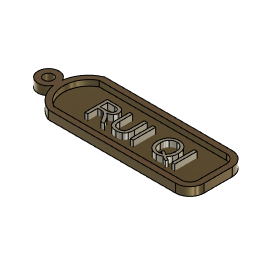
Keychain v1 (Autodesk Fusion 360 design; units mm, degrees)
Autodesk Fusion 360 part; units mm, degrees
sketch "Sketch1" plane through (0, 0, 0) normal (0, 0, 1) x (1, 0, 0) in component "Component"
  line L0 (0, 0) -> (45, 0)
  line L1 (50, 5) -> (50, 15)
  line L2 (45, 20) -> (0, 20)
  arc A0 (50, 15) -> (45, 20) centre (45, 15) ccw
  arc A1 (45, 0) -> (50, 5) centre (45, 5) ccw
  arc A2 (-6.5358, 11.6362) -> (-6.5358, 8.3638) centre (-9.91, 10) ccw
  arc A3 (0, 20) -> (-6.5358, 11.6362) centre (4.1775, 10) ccw
  arc A4 (-6.5358, 8.3638) -> (0, 0) centre (4.1775, 10) ccw
  circle A5 centre (-9.91, 10) radius 1.75
  line L3 (0, 2) -> (45, 2)
  line L4 (48, 5) -> (48, 15)
  line L5 (45, 18) -> (0, 18)
  arc A6 (0, 18) -> (0, 2) centre (4.537, 10) ccw
  arc A7 (45, 2) -> (48, 5) centre (45, 5) ccw
  arc A8 (48, 15) -> (45, 18) centre (45, 15) ccw
  line L6 (7.2298, 5.0727) -> (38.989, 5.0727) construction
  line L7 (38.989, 5.0727) -> (38.989, 16.0727) construction
  line L8 (38.989, 16.0727) -> (7.2298, 16.0727) construction
  line L9 (7.2298, 16.0727) -> (7.2298, 5.0727) construction
  dimension "d4" = 3.5
  dimension "d7" = 2
  text T0 "RUI QI" font "Arial" height 11 align ink ink in box 0 x 0 at (7.2298, 5.0727) x (1, 0) y (0, 1) spacing 1 height is em
  constraint horizontal L0
  constraint vertical L1
  constraint horizontal L2
  constraint coincident L0.start A4.end
  constraint tangent L2 A0
  constraint tangent L1 A1
  constraint coincident A2.end A3
  constraint concentric A3 A4
  constraint concentric A2 A5
  constraint horizontal L3
  constraint vertical L4
  constraint horizontal L5
  constraint concentric A0 A8
  constraint tangent L5 A8
  constraint concentric A1 A7
  constraint tangent L3 A7
  constraint perpendicular L6 L7
  constraint parallel L6 L8
  constraint parallel L7 L9
  measures "d4" diameter of A5
  measures "d7" distance of L0.start L3.start
extrude "Extrude3" add sketch "Sketch1" along normal blind 1 contours L3 L4 L5 A6 A7 A8 makes body 1 in component "Component"
extrude "Extrude1" add sketch "Sketch1" along normal blind 3 separate body makes body 2 in component "Component"
extrude "Extrude2" add sketch "Sketch1" along normal blind 3 separate body text T0 makes body 3 at (15.5309, 10.5479, 0) makes body 4 at (23.2886, 8.3296, 1) makes body 5 at (29.2434, 10.1319, 0) makes body 6 at (37.957, 8.3296, 1) makes body 7 at (7.2398, 8.3296, 1) in component "Component"
component "Component" placed x (1, 0, 0) y (0, 1, 0) z (0, 0, 1) at (0, 0, 0)
